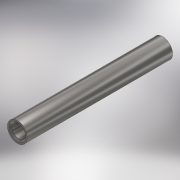
# Autodesk Inventor part: Rod 3-8in
Saved by Autodesk Inventor 2018 (Build 220112000, 112)
## iProperties
Created: 2018-02-12
Part Number: Rod 3-8in
Material: Stainless Steel
Document SubType Name: Modeling
Designer: Moochster
Density: 8 g/cm^3
Appearance: Semi-Polished
Mass: 15.994 g
Surface Area: 26.9907 cm^2
Volume: 1.99925 cm^3
Author: Moochster
Autodesk Inventor part; units mm, degrees
ref_plane "YZ Plane" through (0, 0, 0) normal (1, 0, 0) x (0, 1, 0)
ref_plane "XZ Plane" through (0, 0, 0) normal (0, 1, 0) x (-1, 0, 0)
ref_plane "XY Plane" through (0, 0, 0) normal (0, 0, 1) x (1, 0, 0)
sketch "Sketch1" plane through (0, 0, 0) normal (0, 1, 0) x (-1, 0, 0)
  circle A0 centre (0, 0) radius 3.275
  circle A1 centre (0, 0) radius 4.8
  dimension "d0" = 6.55
  dimension "d1" = 9.6
  constraints: 2 centre point, 2 coincident
  measures "d0" diameter of A0
  measures "d1" diameter of A1
extrude "Extrusion1" add sketch "Sketch1" along normal blind 70
chamfer "Chamfer1" distance 0.75 angle 45 2 edges at (3.275, 70, 0) (3.275, 0, 0)
body "Solid1"
